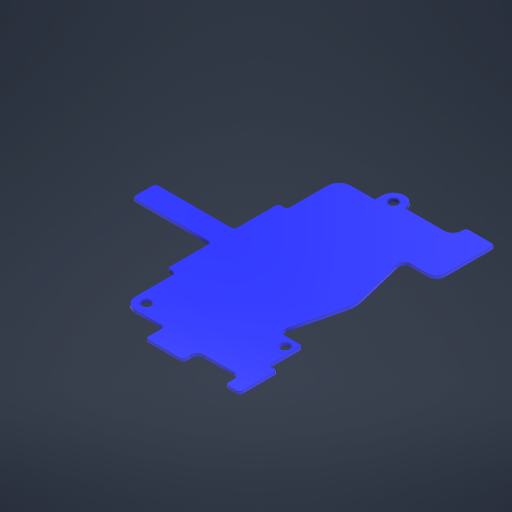
# Autodesk Inventor part: pcb
Saved by Autodesk Inventor 2024 (Build 280153000, 153)
## iProperties
Created: 2024-05-25
Part Number: pcb
Material: Generic
Document SubType Name: Modeling
Designer: Adam
Density: 1 g/cm^3
Appearance: Default
Author: Adam
Autodesk Inventor part; units mm, degrees
ref_plane "YZ Plane" through (0, 0, 0) normal (1, 0, 0) x (0, 1, 0)
ref_plane "XZ Plane" through (0, 0, 0) normal (0, 1, 0) x (-1, 0, 0)
ref_plane "XY Plane" through (0, 0, 0) normal (0, 0, 1) x (1, 0, 0)
ref_plane "Work Plane2" through (0, 1, 0) normal (0, 1, 0) x (1, 0, 0)
sketch "Sketch2" plane through (0, 1, 0) normal (0, 1, 0) x (1, 0, 0)
  arc A0 (-13.8229, -33.4026) -> (-9.8229, -37.4026) centre (-9.8229, -33.4026) ccw
  arc A1 (-9.8229, 36.9551) -> (-13.8229, 32.9551) centre (-9.8229, 32.9551) ccw
  circle A2 centre (2.4699, 39.3408) radius 1.55
  circle A3 centre (26.9336, -22.3933) radius 1.55
  circle A4 centre (-9.8229, -33.4026) radius 1.55
  line L0 (23.7927, 44.0538) -> (31.7927, 44.0538)
  line L1 (32.7927, 43.0538) -> (32.7927, 26.8418)
  line L2 (29.7927, 23.8418) -> (25.2541, 23.8418)
  line L3 (-17.8229, 3.7762) -> (-42.9549, 3.7762)
  line L4 (-43.9549, 2.7762) -> (-43.9549, -3.2238)
  line L5 (-42.9549, -4.2238) -> (-17.8229, -4.2238)
  line L6 (28.7927, -43.9467) -> (31.7927, -43.9467)
  line L7 (22.7927, 43.0538) -> (22.7927, 42.5538)
  arc A5 (23.7927, 44.0538) -> (22.7927, 43.0538) centre (23.7927, 43.0538) ccw
  arc A6 (32.7927, 43.0538) -> (31.7927, 44.0538) centre (31.7927, 43.0538) ccw
  arc A7 (31.7927, -43.9467) -> (32.7927, -42.9467) centre (31.7927, -42.9467) ccw
  arc A8 (27.7927, -42.9467) -> (28.7927, -43.9467) centre (28.7927, -42.9467) ccw
  arc A9 (29.7927, 23.8418) -> (32.7927, 26.8418) centre (29.7927, 26.8418) ccw
  arc A10 (19.7927, 39.5538) -> (22.7927, 42.5538) centre (19.7927, 42.5538) ccw
  arc A11 (-42.9549, 3.7762) -> (-43.9549, 2.7762) centre (-42.9549, 2.7762) ccw
  arc A12 (-43.9549, -3.2238) -> (-42.9549, -4.2238) centre (-42.9549, -3.2238) ccw
  line L8 (-13.8229, 32.9551) -> (-13.8229, 19.9551)
  line L9 (-14.8229, 18.9551) -> (-15.8229, 18.9551)
  line L10 (-16.8229, 17.9551) -> (-16.8229, 4.7762)
  line L11 (-13.8229, -33.4026) -> (-13.8229, -20.4026)
  line L12 (-14.8229, -19.4026) -> (-15.8229, -19.4026)
  line L13 (-16.8229, -18.4026) -> (-16.8229, -5.2238)
  arc A13 (-14.8229, 18.9551) -> (-13.8229, 19.9551) centre (-14.8229, 19.9551) ccw
  arc A14 (-15.8229, 18.9551) -> (-16.8229, 17.9551) centre (-15.8229, 17.9551) ccw
  arc A15 (-17.8229, 3.7762) -> (-16.8229, 4.7762) centre (-17.8229, 4.7762) ccw
  arc A16 (-16.8229, -5.2238) -> (-17.8229, -4.2238) centre (-17.8229, -5.2238) ccw
  arc A17 (-16.8229, -18.4026) -> (-15.8229, -19.4026) centre (-15.8229, -18.4026) ccw
  arc A18 (-13.8229, -20.4026) -> (-14.8229, -19.4026) centre (-14.8229, -20.4026) ccw
  arc A19 (2.4699, 43.3408) -> (-1.5298, 39.3918) centre (2.4699, 39.3408) ccw
  line L14 (-1.5298, 39.3918) -> (-1.5298, 36.9551)
  line L15 (-1.5298, 36.9551) -> (-9.8229, 36.9551)
  line L16 (12.2983, -43.9467) -> (1.2983, -43.9467)
  line L17 (0.2983, -42.9467) -> (0.2983, -38.4026)
  line L18 (-0.7017, -37.4026) -> (-9.8229, -37.4026)
  arc A20 (0.2983, -42.9467) -> (1.2983, -43.9467) centre (1.2983, -42.9467) ccw
  arc A21 (12.2983, -43.9467) -> (13.2983, -42.9467) centre (12.2983, -42.9467) ccw
  arc A22 (0.2983, -38.4026) -> (-0.7017, -37.4026) centre (-0.7017, -38.4026) ccw
  line L19 (19.7927, 39.5538) -> (8.4489, 39.5538)
  line L20 (27.7927, -42.9467) -> (27.7927, -40.9467)
  line L21 (25.7927, -38.9467) -> (15.2983, -38.9467)
  arc A23 (27.7927, -40.9467) -> (25.7927, -38.9467) centre (25.7927, -40.9467) ccw
  line L22 (13.2983, -42.9467) -> (13.2983, -40.9467)
  arc A24 (15.2983, -38.9467) -> (13.2983, -40.9467) centre (15.2983, -40.9467) ccw
  line L23 (8.4489, 39.5538) -> (6.4642, 39.5538)
  arc A25 (6.4642, 39.5538) -> (2.4699, 43.3408) centre (2.4699, 39.3408) ccw
  line L24 (25.2541, -19.1582) -> (28.7927, -19.1582)
  line L25 (28.7927, -19.1582) -> (28.7927, -19.1582)
  line L26 (29.7927, -20.1582) -> (29.7927, -29.8512)
  line L27 (32.7927, -42.9467) -> (32.7927, -31.8512)
  line L28 (31.7927, -30.8512) -> (30.7927, -30.8512)
  arc A26 (29.7927, -20.1582) -> (28.7927, -19.1582) centre (28.7927, -20.1582) ccw
  arc A27 (29.7927, -29.8512) -> (30.7927, -30.8512) centre (30.7927, -29.8512) ccw
  arc A28 (32.7927, -31.8512) -> (31.7927, -30.8512) centre (31.7927, -31.8512) ccw
  line L29 (25.2541, 23.8418) -> (23.8455, 23.8418)
  line L30 (21.9025, 21.3673) -> (25.9693, 4.7141)
  line L31 (25.9693, -0.0306) -> (21.9025, -16.6838)
  line L32 (23.8455, -19.1582) -> (25.7927, -19.1582)
  arc A29 (23.8455, 23.8418) -> (21.9025, 21.3673) centre (23.8455, 21.8418) ccw
  arc A30 (21.9025, -16.6838) -> (23.8455, -19.1582) centre (23.8455, -17.1582) ccw
  arc A31 (25.9693, -0.0306) -> (25.9693, 4.7141) centre (16.2548, 2.3418) ccw
  point P0 (0, 0)
  point P1 (22.7927, 44.0538)
  point P2 (32.7927, 44.0538)
  point P3 (32.7927, 23.8418)
  point P4 (32.7927, -43.9467)
  point P5 (-16.8229, 3.7762)
  point P6 (-16.8229, -4.2238)
  point P7 (21.2983, 23.8418)
  point P8 (30.2927, -43.9467)
  point P9 (-13.8229, 18.9551)
  point P10 (-16.8229, 18.9551)
  point P11 (-13.8229, -19.4026)
  point P12 (-16.8229, -19.4026)
  point P13 (13.2983, -43.9467)
  point P14 (0.2983, -43.9467)
  point P15 (0.2983, -37.4026)
  point P16 (27.7927, -38.9467)
  point P17 (27.7927, -42.9467)
  point P18 (29.7927, -19.1582)
  point P19 (27.0234, -19.1582)
  point P20 (27.5234, 23.8418)
  point P21 (26.5486, 2.3418)
  dimension "d13" = 3.1
  dimension "d15" = 3.1
  dimension "d26" = 1
  dimension "d27" = 3
  dimension "d32" = 1
  dimension "d33" = 20.212
  dimension "d36" = 14
  dimension "d37" = 3
  dimension "d38" = 14
  dimension "d39" = 3
  dimension "d40" = 1
  dimension "d42" = 13
  dimension "d43" = 1
  dimension "d47" = 88.0005
  dimension "d49" = 4
  dimension "d50" = 2
  dimension "d51" = 2
  dimension "d52" = 0.5
  dimension "d57" = 1
  dimension "d58" = 43
  dimension "d60" = 21.5
  dimension "d61" = 2
  dimension "d62" = 10
  constraints: 66 end point, 58 point on circle, 47 tangent, 35 point on line, 32 centre point, 15 equal radius, 12 perpendicular, 7 vertical, 6 horizontal, 3 midpoint, 2 coincident
  measures "d13" diameter of A2
  measures "d15" diameter of A4
  measures "d26" radius of A5
  measures "d27" radius of A9
  measures "d32" radius of A11
  measures "d33" distance between parallel lines of L2 L0
  measures "d36" distance of L8.start point (-13.823, 18.955)
  measures "d37" distance of point (-13.823, 18.955) point (-16.823, 18.955)
  measures "d38" distance of L11.start point (-13.823, -19.403)
  measures "d39" distance between parallel lines of L11 L13
  measures "d40" radius of A13
  measures "d42" distance of point (13.298, -43.947) point (0.298, -43.947)
  measures "d43" radius of A20
  measures "d47" distance between parallel lines of L6 L0
  measures "d49" distance of L20.start point (27.793, -38.947)
  measures "d50" radius of A23
  measures "d51" radius of A24
  measures "d52" distance of L7.start L7.end
  measures "d57" radius of A26
  measures "d58" vertical distance of point (27.023, -19.158) point (27.523, 23.842)
  measures "d60" distance from line of point (26.549, 2.342) L24
  measures "d61" radius of A29
  measures "d62" radius of A31
extrude "Extrusion2" add sketch "Sketch2" along normal blind 1
body "Solid2"
